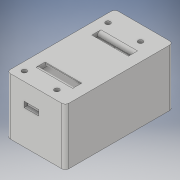
# Autodesk Inventor part: bottom
Saved by Autodesk Inventor 2017.3 (Build 213257000, 257)
## iProperties
Part Number: bottom
Material: Generisch
Document SubType Name: Modeling
Designer: Enno
Density: 1 g/cm^3
Appearance: Vorgabe
Author: Enno
Autodesk Inventor part; units mm, degrees
ref_plane "YZ Plane" through (0, 0, 0) normal (1, 0, 0) x (0, 1, 0)
ref_plane "XZ Plane" through (0, 0, 0) normal (0, 1, 0) x (-1, 0, 0)
ref_plane "XY Plane" through (0, 0, 0) normal (0, 0, 1) x (1, 0, 0)
sketch "Skizze1" plane through (0, 0, 0) normal (0, 0, 1) x (1, 0, 0)
  line L0 (0, 0) -> (32, 0)
  line L1 (32, 0) -> (32, 59)
  line L2 (32, 59) -> (0, 59)
  line L3 (0, 59) -> (0, 0)
  dimension "d0" = 32
  dimension "d1" = 59
  constraints: 8 end point, 2 parallel, 1 horizontal, 1 perpendicular
  measures "d0" distance of L1.end L2.end
  measures "d1" distance of L0.end L1.end
extrude "Extrusion1" add sketch "Skizze1" against normal blind 31
sketch "Skizze2" plane through (0, 0, -31) normal (0, 0, -1) x (-1, 0, 0)
  line L0 (-2, 57) -> (-30, 57)
  line L1 (-30, 57) -> (-30, 2)
  line L2 (-30, 2) -> (-2, 2)
  line L3 (-2, 2) -> (-2, 57)
  line L4 (0, 59) -> (-32, 59) construction
  line L5 (-32, 59) -> (-32, 0) construction
  point P0 (0, 0)
  dimension "d4" = 2
  dimension "d5" = 2
  dimension "d6" = 2
  dimension "d7" = 2
  constraints: 8 end point, 2 parallel, 1 horizontal, 1 perpendicular
  measures "d4" distance from line of point (0, 0) L2
  measures "d5" distance from line of point (0, 0) L3
  measures "d6" distance from line of L4 L0.start
  measures "d7" distance from line of L5 L0.end
extrude "Extrusion2" cut sketch "Skizze2" against normal blind 28.5
sketch "Skizze8" plane through (0, 0, -2.5) normal (0, 0, -1) x (-1, 0, 0)
  line L0 (-6, 12) -> (-26, 12)
  line L1 (-26, 12) -> (-26, 15)
  line L2 (-26, 15) -> (-6, 15)
  line L3 (-6, 15) -> (-6, 12)
  line L4 (-2, 2) -> (-30, 2) construction
  circle A0 centre (-4.61, 4.57) radius 3 construction
  line L5 (-6, 43.5) -> (-26, 43.5)
  line L6 (-26, 43.5) -> (-26, 40.5)
  line L7 (-26, 40.5) -> (-6, 40.5)
  line L8 (-6, 40.5) -> (-6, 43.5)
  circle A1 centre (-4.61, 50.29) radius 3 construction
  line L9 (-30, 57) -> (-2, 57) projected
  point P0 (0, 0)
  point P1 (-16, 12)
  point P2 (-16, 2)
  point P3 (-16, 2)
  point P4 (-16, 40.5)
  dimension "d43" = 3
  dimension "d44" = 20
  dimension "d46" = 3
  dimension "d47" = 20
  dimension "d71" = 10
  dimension "d72" = 13.5
  constraints: 16 end point, 4 midpoint, 4 parallel, 2 horizontal, 2 perpendicular, 2 vertical alignment
  measures "d43" distance of L2.end L0.start
  measures "d44" distance of L0.start L0.end
  measures "d46" distance of L7.end L5.start
  measures "d47" distance of L6.end L7.end
  measures "d71" distance between parallel lines of L4 L0
  measures "d72" distance between parallel lines of L9 L5
extrude "Extrusion5" cut sketch "Skizze8" against normal through all
sketch "Skizze9" plane through (0, 0, 0) normal (0, -1, 0) x (1, 0, 0)
  line L0 (2, -5.5) -> (3.0624, -5.5) construction
  line L1 (17.5, -12.3) -> (9.5, -12.3)
  line L2 (9.5, -12.3) -> (9.5, -9.3)
  line L3 (9.5, -9.3) -> (17.5, -9.3)
  line L4 (17.5, -9.3) -> (17.5, -12.3)
  line L5 (0, 0) -> (32, 0) construction
  line L6 (2, -2.5) -> (30, -2.5) projected
  line L7 (2, -31) -> (2, -2.5) projected
  point P0 (13.5, -9.3)
  point P1 (16, 0)
  point P2 (6.1576, -2)
  point P3 (20.8424, -2)
  point P4 (30, -2.5)
  dimension "d54" = 8
  dimension "d55" = 3
  dimension "d70" = 6.8
  dimension "d81" = 7.5
  constraints: 8 end point, 2 midpoint, 2 parallel, 1 horizontal, 1 perpendicular, 1 other
  measures "d54" distance of L2.end L3.end
  measures "d55" distance of L1.end L2.end
  measures "d81" distance between parallel lines of L7 L2
extrude "Extrusion6" cut sketch "Skizze9" against normal up to surface (2 mm away)
fillet "Rundung1" radius 2 4 edges at (32, 0, -15.5) (0, 0, -15.5) (0, 59, -15.5) (32, 59, -15.5)
fillet "Rundung2" radius 2 2 edges at (16, 15, -2.5) (16, 40.5, -2.5)
fillet "Rundung3" radius 2 2 edges at (16, 12, 0) (16, 43.5, 0)
sketch "Skizze11" plane through (0, 0, -2.5) normal (0, 0, -1) x (-1, 0, 0)
  point P0 (0, 0)
  point P1 (-22.39, 5)
  point P2 (-22.39, 5)
  point P3 (-4.61, 5)
  point P4 (-4.61, 5)
  point P5 (-22.39, 50.72)
  point P6 (-22.39, 50.72)
  point P7 (-4.61, 50.72)
  dimension "d82" = 4.61
  dimension "d83" = 5
  dimension "d84" = 45.72
  dimension "d85" = 17.78
  constraints: 4 coincident, 2 horizontal alignment, 2 vertical alignment
  measures "d82" horizontal distance of point (0, 0) point (-4.61, 5)
  measures "d83" vertical distance of point (0, 0) point (-4.61, 5)
  measures "d84" distance of point (-4.61, 5) point (-4.61, 50.72)
  measures "d85" distance of point (-4.61, 50.72) point (-22.39, 50.72)
hole "Bohrung4" at (22.39, 5, -2.5) at (4.61, 5, -2.5) at (22.39, 50.72, -2.5) at (4.61, 50.72, -2.5) direction (0, 0, 1) diameter 2.6 end through all
